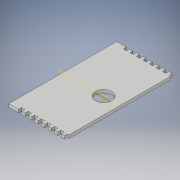
# Autodesk Inventor part: Side_two
Saved by Autodesk Inventor 2019.4 (Build 234330000, 330)
## iProperties
Created: 2019-12-17
Part Number: Side_two
Material: Generic
Document SubType Name: Modeling
Designer: fabfarm
Density: 1 g/cm^3
Appearance: Default
Author: fabfarm
Autodesk Inventor part; units mm, degrees
ref_plane "YZ Plane" through (0, 0, 0) normal (1, 0, 0) x (0, 1, 0)
ref_plane "XZ Plane" through (0, 0, 0) normal (0, 1, 0) x (-1, 0, 0)
ref_plane "XY Plane" through (0, 0, 0) normal (0, 0, 1) x (1, 0, 0)
sketch "Sketch1" plane through (0, 0, 0) normal (0, 1, 0) x (-1, 0, 0)
  line L0 (0, 0) -> (350, 0)
  line L1 (350, 0) -> (350, 660)
  line L2 (350, 660) -> (0, 660)
  line L3 (0, 660) -> (0, 0)
  dimension "d0" = 350
  dimension "d1" = 660
  constraints: 8 end point, 2 parallel, 1 horizontal, 1 perpendicular
  measures "d0" distance of L0.start L0.end
  measures "d1" distance of L2.end L0.start
extrude "Extrusion1" add sketch "Sketch1" along normal blind 18.55
sketch "Sketch2" plane through (0, 18.55, 0) normal (0, 1, 0) x (1, 0, 0)
  line L0 (-290, -641.45) -> (-270, -641.45)
  line L1 (-270, -641.45) -> (-270, -660)
  line L2 (-270, -660) -> (-290, -660)
  line L3 (-290, -660) -> (-290, -641.45)
  line L4 (-350, -660) -> (0, -660) projected
  line L5 (-350, 0) -> (-350, -660) projected
  line L6 (-250, -641.45) -> (-230, -641.45)
  line L7 (-230, -641.45) -> (-230, -660)
  line L8 (-250, -660) -> (-250, -641.45)
  line L9 (-230, -660) -> (-250, -660)
  line L10 (-210, -641.45) -> (-190, -641.45)
  line L11 (-190, -641.45) -> (-190, -660)
  line L12 (-210, -660) -> (-210, -641.45)
  line L13 (-190, -660) -> (-210, -660)
  line L14 (-170, -641.45) -> (-150, -641.45)
  line L15 (-150, -641.45) -> (-150, -660)
  line L16 (-170, -660) -> (-170, -641.45)
  line L17 (-150, -660) -> (-170, -660)
  line L18 (-130, -641.45) -> (-110, -641.45)
  line L19 (-110, -641.45) -> (-110, -660)
  line L20 (-130, -660) -> (-130, -641.45)
  line L21 (-110, -660) -> (-130, -660)
  line L22 (-90, -641.45) -> (-70, -641.45)
  line L23 (-70, -641.45) -> (-70, -660)
  line L24 (-90, -660) -> (-90, -641.45)
  line L25 (-70, -660) -> (-90, -660)
  line L26 (-50, -641.45) -> (-30, -641.45)
  line L27 (-30, -641.45) -> (-30, -660)
  line L28 (-50, -660) -> (-50, -641.45)
  line L29 (-30, -660) -> (-50, -660)
  point P0 (0, 0)
  dimension "d4" = 18.55
  dimension "d5" = 20
  dimension "d6" = 60
  dimension "d9" = 40
  constraints: 56 end point, 2 horizontal, 2 parallel, 1 collinear, 1 perpendicular, 48 other
  measures "d4" distance of L0.end L1.end
  measures "d5" distance of L0.start L0.end
  measures "d6" distance between parallel lines of L5 L3
  measures "d9" distance of L0.start L6.start
ref_plane "Work Plane1" through (-350, 0, 330) normal (0, 0, 1) x (1, 0, 0)
extrude "Extrusion2" cut sketch "Sketch2" against normal blind 18.55
sketch "Sketch3" plane through (0, 18.55, 0) normal (0, 1, 0) x (1, 0, 0)
  line L0 (-50, -641.45) -> (-30, -641.45) projected
  line L1 (-10, -660) -> (0, -660)
  line L2 (0, -660) -> (0, -641.45)
  line L3 (0, -641.45) -> (-10, -641.45)
  line L4 (-10, -641.45) -> (-10, -660)
  line L5 (-30, -660) -> (0, -660) projected
  line L6 (-30, -641.45) -> (-30, -660) projected
  line L7 (0, -660) -> (0, 0) projected
  dimension "d17" = 20
  constraints: 8 end point, 3 collinear, 2 parallel, 1 horizontal, 1 perpendicular
  measures "d17" distance between parallel lines of L6 L4
extrude "Extrusion3" cut sketch "Sketch3" against normal blind 18.55
mirror "Mirror1" about plane through (-350, 0, 330) normal (0, 0, 1) of "Extrusion2", "Extrusion3"
sketch "Sketch4" plane through (0, 18.55, 0) normal (0, 1, 0) x (1, 0, 0)
  circle A0 centre (-100, -330) radius 50
  line L0 (70, -330) -> (-420, -330) projected
  line L1 (0, -641.45) -> (0, -18.55) projected
  point P0 (0, 0)
  dimension "d20" = 100
  dimension "d21" = 100
  constraints: 1 centre point, 1 point on line
  measures "d20" diameter of A0
  measures "d21" distance from line of L1 A0.centre
extrude "Extrusion4" cut sketch "Sketch4" against normal blind 20
body "Solid1"
